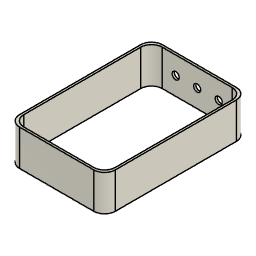
Connector v2 (Autodesk Fusion 360 design; units mm, degrees)
Autodesk Fusion 360 part; units mm, degrees
sketch "Sketch1" plane through (0, 0, 0) normal (0, 0, 1) x (1, 0, 0)
  line L0 (51.75, -99.5) -> (-51.75, -99.5)
  line L1 (-66.75, -84.5) -> (-66.75, 84.5)
  line L2 (-51.75, 99.5) -> (51.75, 99.5)
  line L3 (66.75, 84.5) -> (66.75, -84.5)
  line L4 (66.75, -99.5) -> (-66.75, 99.5) construction
  line L5 (-66.75, -99.5) -> (66.75, 99.5) construction
  line L6 (48.75, 96.5) -> (-48.75, 96.5)
  line L7 (-63.75, 81.5) -> (-63.75, -81.5)
  line L8 (-48.75, -96.5) -> (48.75, -96.5)
  line L9 (63.75, -81.5) -> (63.75, 81.5)
  line L10 (63.75, 96.5) -> (-63.75, -96.5) construction
  line L11 (-63.75, 96.5) -> (63.75, -96.5) construction
  arc A0 (-63.75, -81.5) -> (-48.75, -96.5) centre (-48.75, -81.5) ccw
  arc A1 (-66.75, -84.5) -> (-51.75, -99.5) centre (-51.75, -84.5) ccw
  arc A2 (48.75, -96.5) -> (63.75, -81.5) centre (48.75, -81.5) ccw
  arc A3 (51.75, -99.5) -> (66.75, -84.5) centre (51.75, -84.5) ccw
  arc A4 (63.75, 81.5) -> (48.75, 96.5) centre (48.75, 81.5) ccw
  arc A5 (66.75, 84.5) -> (51.75, 99.5) centre (51.75, 84.5) ccw
  arc A6 (-51.75, 99.5) -> (-66.75, 84.5) centre (-51.75, 84.5) ccw
  arc A7 (-48.75, 96.5) -> (-63.75, 81.5) centre (-48.75, 81.5) ccw
  dimension "d1" = 133.5
  dimension "d2" = 199
  dimension "d3" = 127.5
  dimension "d4" = 193
  dimension "d5" = 15
  dimension "d6" = 15
  dimension "d7" = 15
  dimension "d8" = 15
  dimension "d9" = 15
  dimension "d10" = 15
  dimension "d11" = 15
  dimension "d12" = 15
  constraint horizontal L0
  constraint perpendicular L0 L1
  constraint parallel L0 L2
  constraint parallel L1 L3
  constraint coincident L4 origin
  constraint coincident L5 origin
  constraint horizontal L6
  constraint perpendicular L6 L7
  constraint parallel L6 L8
  constraint parallel L7 L9
  constraint coincident L10 origin
  constraint coincident L11 origin
  constraint coincident L10.end L7
  constraint coincident L10.end L8
  constraint tangent L7 A0
  constraint tangent L8 A0
  constraint coincident L5.start L1
  constraint coincident L5.start L0
  constraint tangent L1 A1
  constraint tangent L0 A1
  constraint coincident L11.end L8
  constraint coincident L11.end L9
  constraint tangent L8 A2
  constraint tangent L9 A2
  constraint coincident L4.start L3
  constraint coincident L4.start L0
  constraint tangent L3 A3
  constraint tangent L0 A3
  constraint coincident L10.start L9
  constraint coincident L10.start L6
  constraint tangent L9 A4
  constraint tangent L6 A4
  constraint coincident L5.end L2
  constraint coincident L5.end L3
  constraint tangent L2 A5
  constraint tangent L3 A5
  constraint coincident L4.end L1
  constraint coincident L4.end L2
  constraint tangent L1 A6
  constraint tangent L2 A6
  constraint coincident L11.start L6
  constraint coincident L11.start L7
  constraint tangent L6 A7
  constraint tangent L7 A7
  measures "d1" distance of L4.end L5.end
  measures "d2" distance of L5.start L4.end
  measures "d3" distance of L10.end L11.end
  measures "d4" distance of L11.start L10.end
  measures "d5" radius of A0
  measures "d6" radius of A1
  measures "d7" radius of A2
  measures "d8" radius of A3
  measures "d9" radius of A4
  measures "d10" radius of A5
  measures "d11" radius of A6
  measures "d12" radius of A7
extrude "Extrude1" add sketch "Sketch1" along normal blind 10
extrude "Extrude2" add 1 faces at (65.75, -27.1667, 10) along direction (0, 0, 1) blind 10
extrude "Extrude3" add 1 faces at (65.75, -27.1667, 20) along direction (0, 0, 1) blind 30
sketch "Sketch2" plane through (0, 99.5, 0) normal (0, 1, 0) x (-1, 0, 0)
  line L0 (-51.75, 0) -> (51.75, 0)
  line L1 (51.75, 0) -> (51.75, 50)
  line L2 (51.75, 50) -> (-51.75, 50)
  line L3 (-51.75, 50) -> (-51.75, 0)
  circle A0 centre (0, 25) radius 5
  circle A1 centre (30, 25) radius 5
  circle A2 centre (-30, 25) radius 5
  dimension "d19" = 10
  dimension "d20" = 10
  dimension "d21" = 10
  measures "d19" diameter of A0
  measures "d20" diameter of A1
  measures "d21" diameter of A2
extrude "Extrude4" cut sketch "Sketch2" against normal blind 10 contours A0 | A1 | A2
